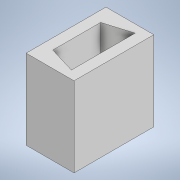
# Autodesk Inventor part: reed-switch-design-test
Saved by Autodesk Inventor 2021 (Build 250183000, 183)
## iProperties
Created: 2021-01-14
Part Number: reed-switch-design-test
Material: Generic
Document SubType Name: Modeling
Designer: Luke Kamols
Density: 1 g/cm^3
Appearance: Default
Author: Luke Kamols
Autodesk Inventor part; units mm, degrees
ref_plane "YZ Plane" through (0, 0, 0) normal (1, 0, 0) x (0, 1, 0)
ref_plane "XZ Plane" through (0, 0, 0) normal (0, 1, 0) x (-1, 0, 0)
ref_plane "XY Plane" through (0, 0, 0) normal (0, 0, 1) x (1, 0, 0)
sketch "Sketch1" plane through (0, 0, 0) normal (0, 1, 0) x (-1, 0, 0)
  line L0 (0, 0) -> (15, 0)
  line L1 (15, 0) -> (15, -15)
  line L2 (15, -15) -> (0, -15)
  line L3 (0, -15) -> (0, 0)
  line L4 (0, 0) -> (3, 0)
  line L5 (3, 0) -> (3, -15)
  line L6 (15, 0) -> (12, 0)
  line L7 (12, 0) -> (12, -15)
  dimension "d0" = 15
  dimension "d1" = 15
  dimension "d11" = 3
  dimension "d12" = 3
  constraints: 16 end point, 4 point on line, 3 perpendicular, 2 parallel, 1 horizontal
  measures "d0" distance of L1.end L2.end
  measures "d1" distance of L0.end L1.end
  measures "d11" distance of L0.start L4.end
  measures "d12" distance of L0.end L6.end
extrude "Extrusion1" add sketch "Sketch1" along normal blind 15 contours L0 L7 L2 L5
sketch "Sketch2" plane through (0, 15, 0) normal (0, 1, 0) x (1, 0, 0)
  line L0 (-3, 15) -> (-12, 15) projected
  line L1 (-15, 15) -> (-15, 0) projected
  line L2 (-7.5, 12) -> (-3, 12)
  line L3 (-3, 12) -> (-3, 3)
  line L4 (-3, 3) -> (-12, 3)
  line L5 (-12, 3) -> (-12, 12)
  line L6 (-12, 12) -> (-7.5, 12)
  line L7 (-7.5, 3) -> (-10, 3)
  line L8 (-10, 3) -> (-10, 12)
  line L9 (-7.5, 3) -> (-5, 3)
  line L10 (-5, 3) -> (-5, 12)
  line L11 (-5, 12) -> (-5, 13.5)
  line L12 (-5, 13.5) -> (-10, 12)
  line L13 (-5, 3) -> (-5, 1.5)
  line L14 (-5, 1.5) -> (-10, 3)
  point P0 (0, 0)
  point P1 (0, 15)
  dimension "d5" = 2.5
  dimension "d6" = 2.5
  dimension "d9" = 1.5
  dimension "d10" = 1.5
  constraints: 26 end point, 5 point on line, 4 perpendicular, 2 vertical, 1 midpoint
  measures "d5" distance of L7.start L7.end
  measures "d6" distance of L7.start L9.end
  measures "d9" distance of L10.end L11.end
  measures "d10" distance of L9.end L13.end
extrude "Extrusion2" cut sketch "Sketch2" against normal blind 13 contours L6 L12 L11 L2 | L2 L10 L4 L8 L6 | L13 L14 L4
chamfer "Chamfer1" distance 5 angle 15 1 edges at (-10, 2, -7.5) measured on face at (-9.5, 2, -7.5)
body "Solid1"
